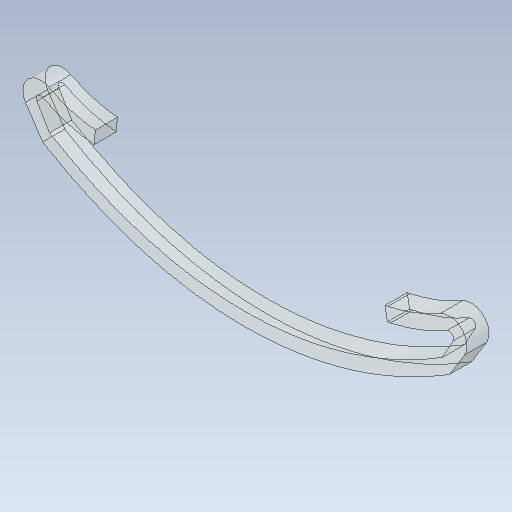
# Autodesk Inventor part: 脚ゴム
Saved by Autodesk Inventor 2020 (Build 240168000, 168)
## iProperties
Created: 2019-11-12
Part Number: 脚ゴム
Material: ゴム、シリコーン
Document SubType Name: Modeling
Designer: tanjihayato
Density: 1.25 g/cm^3
Appearance: クリア
Mass: 2.72773 g
Surface Area: 23.6428 cm^2
Volume: 2.18218 cm^3
Author: tanjihayato
Autodesk Inventor part; units mm, degrees
ref_plane "YZ Plane" through (0, 0, 0) normal (1, 0, 0) x (0, 1, 0)
ref_plane "XZ Plane" through (0, 0, 0) normal (0, 1, 0) x (-1, 0, 0)
ref_plane "XY Plane" through (0, 0, 0) normal (0, 0, 1) x (1, 0, 0)
sketch "スケッチ1" plane through (0, 0, 0) normal (0, 0, 1) x (1, 0, 0)
  arc A0 (47.1325, -53.2266) -> (45.758, -51.8784) centre (46.2557, -52.7457) ccw
  arc A1 (33.009, -56.7784) -> (45.758, -51.8784) centre (23.6069, -13.28) ccw
  arc A2 (11.1932, -28.6204) -> (33.009, -56.7784) centre (28.8377, -37.4801) ccw
  arc A3 (11.1932, -28.6204) -> (-11.1841, -28.6384) centre (0, -23) ccw
  arc A4 (-22.0046, -54.1258) -> (-11.1841, -28.6384) centre (-27.3796, -36.8033) ccw
  arc A5 (-45.6895, -51.9306) -> (-22.0046, -54.1258) centre (-31.2017, -24.4856) ccw
  arc A6 (-45.6895, -51.9306) -> (-47.014, -53.3291) centre (-46.1563, -52.815) ccw
  line L0 (-47.014, -53.3291) -> (-44.145, -58.1151)
  spline S0 degree 4 poles (-44.145, -58.1151) (-43.8381, -58.3003) (-43.4088, -58.5568) (-42.8575, -58.8816) (-42.1841, -59.2711) (-41.6963, -59.5497) (-41.2094, -59.8243) (-40.7232, -60.0949) (-40.2377, -60.3617) (-39.7528, -60.6247) (-39.2684, -60.8839) (-38.7844, -61.1395) (-38.3007, -61.3914) (-37.8172, -61.6398) (-37.334, -61.8846) (-36.8508, -62.1259) (-36.3678, -62.3637) (-35.8847, -62.5981) (-35.4015, -62.8291) (-34.9183, -63.0567) (-34.4349, -63.281) (-33.9513, -63.502) (-33.4675, -63.7196) (-32.9834, -63.934) (-32.499, -64.1451) (-32.0143, -64.3529) (-31.5292, -64.5576) (-31.0437, -64.7589) (-30.5578, -64.9571) (-30.0715, -65.1521) (-29.5847, -65.3439) (-29.0974, -65.5325) (-28.6097, -65.7179) (-28.1214, -65.9001) (-27.6326, -66.0792) (-27.1433, -66.2551) (-26.6534, -66.4278) (-26.163, -66.5974) (-25.6721, -66.7638) (-25.1806, -66.927) (-24.6885, -67.0871) (-24.1958, -67.244) (-23.7026, -67.3978) (-23.2087, -67.5484) (-22.7144, -67.6958) (-22.2194, -67.8401) (-21.7238, -67.9811) (-21.2277, -68.1191) (-20.7311, -68.2538) (-20.2338, -68.3854) (-19.736, -68.5137) (-19.2377, -68.6389) (-18.7388, -68.7609) (-18.2393, -68.8798) (-17.7394, -68.9954) (-17.2389, -69.1078) (-16.7379, -69.217) (-16.2363, -69.323) (-15.7343, -69.4258) (-15.2318, -69.5254) (-14.7289, -69.6218) (-14.2255, -69.7149) (-13.7216, -69.8049) (-13.2173, -69.8915) (-12.7125, -69.975) (-12.2074, -70.0552) (-11.7018, -70.1322) (-11.1959, -70.2059) (-10.6896, -70.2764) (-10.1829, -70.3436) (-9.6759, -70.4075) (-9.1686, -70.4683) (-8.661, -70.5257) (-8.1531, -70.5799) (-7.6449, -70.6308) (-7.1364, -70.6784) (-6.6277, -70.7228) (-6.1188, -70.7639) (-5.6096, -70.8017) (-5.1003, -70.8362) (-4.5907, -70.8674) (-4.0811, -70.8954) (-3.5712, -70.9201) (-3.0613, -70.9415) (-2.5513, -70.9596) (-2.0411, -70.9744) (-1.5309, -70.9859) (-1.0206, -70.9941) (-0.5103, -70.9991) (0, -71.0007) (0.5103, -70.9991) (1.0206, -70.9941) (1.5309, -70.9859) (2.0411, -70.9744) (2.5512, -70.9596) (3.0613, -70.9415) (3.5712, -70.9201) (4.0811, -70.8954) (4.5907, -70.8674) (5.1002, -70.8362) (5.6096, -70.8017) (6.1187, -70.7639) (6.6276, -70.7228) (7.1363, -70.6784) (7.6447, -70.6308) (8.1529, -70.5799) (8.6608, -70.5257) (9.1683, -70.4683) (9.6756, -70.4076) (10.1825, -70.3436) (10.6891, -70.2764) (11.1953, -70.2059) (11.7011, -70.1322) (12.2065, -70.0553) (12.7115, -69.9751) (13.2161, -69.8917) (13.7202, -69.805) (14.2238, -69.7151) (14.727, -69.622) (15.2297, -69.5257) (15.7318, -69.4261) (16.2335, -69.3234) (16.7346, -69.2175) (17.2352, -69.1083) (17.7352, -68.996) (18.2346, -68.8805) (18.7335, -68.7617) (19.2317, -68.6399) (19.7293, -68.5148) (20.2264, -68.3866) (20.7227, -68.2552) (21.2185, -68.1207) (21.7136, -67.983) (22.208, -67.8421) (22.7018, -67.6981) (23.1948, -67.551) (23.6872, -67.4008) (24.1789, -67.2474) (24.6699, -67.0909) (25.1602, -66.9313) (25.6497, -66.7686) (26.1386, -66.6028) (26.6267, -66.4339) (27.1141, -66.2618) (27.6008, -66.0867) (28.0867, -65.9085) (28.5719, -65.7272) (29.0563, -65.5428) (29.54, -65.3554) (30.023, -65.1648) (30.5052, -64.9712) (30.9867, -64.7745) (31.4674, -64.5748) (31.9475, -64.3719) (32.4267, -64.166) (32.9053, -63.9571) (33.3831, -63.745) (33.8603, -63.5299) (34.3367, -63.3117) (34.8124, -63.0904) (35.2875, -62.8661) (35.7619, -62.6386) (36.2356, -62.4081) (36.7086, -62.1745) (37.181, -61.9378) (37.6528, -61.698) (38.124, -61.455) (38.5946, -61.209) (39.0646, -60.9598) (39.5341, -60.7075) (40.003, -60.452) (40.4714, -60.1934) (40.9394, -59.9316) (41.4069, -59.6666) (41.8739, -59.3984) (42.3406, -59.127) (42.8069, -58.8523) (43.4481, -58.4698) (43.9715, -58.1517) (44.3779, -57.9011) (44.6679, -57.7205) knots 0 0 0 0 0 0.014541 0.020333 0.02611 0.031872 0.03762 0.043355 0.049078 0.054789 0.060489 0.066178 0.071857 0.077527 0.083187 0.088839 0.094483 0.10012 0.105749 0.111371 0.116986 0.122595 0.128199 0.133797 0.139389 0.144976 0.150559 0.156136 0.16171 0.167279 0.172845 0.178407 0.183965 0.18952 0.195072 0.20062 0.206166 0.211709 0.21725 0.222788 0.228323 0.233857 0.239388 0.244918 0.250445 0.255971 0.261495 0.267017 0.272538 0.278057 0.283575 0.289092 0.294608 0.300122 0.305635 0.311147 0.316658 0.322169 0.327678 0.333186 0.338694 0.344201 0.349707 0.355213 0.360718 0.366222 0.371726 0.377229 0.382732 0.388235 0.393737 0.399238 0.404739 0.41024 0.415741 0.421241 0.426741 0.432241 0.43774 0.44324 0.448739 0.454238 0.459737 0.465236 0.470734 0.476233 0.481731 0.48723 0.492728 0.498227 0.503725 0.509224 0.514722 0.520221 0.525719 0.531218 0.536717 0.542216 0.547715 0.553214 0.558714 0.564214 0.569713 0.575214 0.580714 0.586215 0.591716 0.597217 0.602718 0.60822 0.613723 0.619225 0.624728 0.630232 0.635736 0.641241 0.646746 0.652251 0.657758 0.663264 0.668772 0.67428 0.679789 0.685299 0.690809 0.69632 0.701832 0.707345 0.712859 0.718374 0.72389 0.729407 0.734925 0.740444 0.745965 0.751487 0.75701 0.762535 0.768061 0.773588 0.779117 0.784648 0.790181 0.795715 0.801252 0.80679 0.812331 0.817873 0.823418 0.828965 0.834515 0.840067 0.845622 0.85118 0.85674 0.862304 0.867871 0.873441 0.879014 0.884591 0.890172 0.895757 0.901345 0.906938 0.912535 0.918137 0.923743 0.929355 0.934971 0.940593 0.946221 0.951854 0.957493 0.963139 0.968791 0.974449 0.980115 0.985788 1 1 1 1 1
  line L1 (44.6679, -57.7205) -> (47.1325, -53.2266)
  arc A7 (4.5969, -37.0887) -> (23.8174, -61.1986) centre (28.8377, -37.4801) ccw
  spline S1 degree 3 poles (23.923, -63.1268) (24.0467, -63.086) (24.1612, -63.0216) (24.3592, -62.8523) (24.4407, -62.7492) (24.5595, -62.5175) (24.5958, -62.3911) (24.6178, -62.1316) (24.6033, -62.0009) (24.5251, -61.7525) (24.4622, -61.6371) (24.3075, -61.4513) (24.2222, -61.3781) (24.0311, -61.2629) (23.9266, -61.2217) (23.8174, -61.1986) knots 0 0 0 0 0.148947 0.148947 0.297893 0.297893 0.44684 0.44684 0.595787 0.595787 0.744733 0.744733 0.872367 0.872367 1 1 1 1
  spline S2 degree 3 poles (23.923, -63.1268) (23.6264, -63.2244) (21.6991, -63.8462) (18.9298, -64.6237) (14.7719, -65.5721) (11.4157, -66.1631) (7.1944, -66.6887) (3.8013, -66.9375) (-0.4475, -67.0324) (-3.8473, -66.9351) (-8.0854, -66.5978) (-11.4616, -66.156) (-15.6527, -65.3916) (-18.978, -64.6118) (-23.0925, -63.431) (-25.7434, -62.5289) (-27.5645, -61.8359) (-27.7718, -61.756) knots -0.770978 -0.770978 -0.770978 -0.770978 -0.760435 -0.70257 -0.673637 -0.615772 -0.58684 -0.528974 -0.500042 -0.442177 -0.413244 -0.355379 -0.326446 -0.268581 -0.239649 -0.181783 -0.174342 -0.174342 -0.174342 -0.174342
  spline S3 degree 3 poles (-27.5161, -59.8282) (-27.6456, -59.8417) (-27.7712, -59.8804) (-28.0006, -60.0037) (-28.1022, -60.0872) (-28.2675, -60.2884) (-28.3298, -60.4042) (-28.4064, -60.6531) (-28.42, -60.7838) (-28.3964, -61.0432) (-28.3594, -61.1693) (-28.2435, -61.3919) (-28.1687, -61.4881) (-27.9885, -61.6491) (-27.8845, -61.7126) (-27.7718, -61.756) knots 0 0 0 0 0.145866 0.145866 0.291731 0.291731 0.437597 0.437597 0.583462 0.583462 0.729328 0.729328 0.864664 0.864664 1 1 1 1
  arc A8 (-27.5161, -59.8282) -> (-20.671, -58.4236) centre (-31.2017, -24.4856) ccw
  arc A9 (-20.671, -58.4236) -> (-4.7434, -37.0245) centre (-27.3796, -36.8033) ccw
  arc A10 (-3.4858, -36.0681) -> (-4.7434, -37.0245) centre (-3.7435, -37.0343) ccw
  arc A11 (-3.4858, -36.0681) -> (3.3494, -36.1037) centre (0, -23) ccw
  arc A12 (4.5969, -37.0887) -> (3.3494, -36.1037) centre (3.597, -37.0726) ccw
  circle A13 centre (0, -23) radius 8.525
  circle A14 centre (0, 0) radius 1.5
  circle A15 centre (-6.3066, -8.8137) radius 1.5
  line L2 (5.2372, 1.6799) -> (11.9265, -19.1744)
  arc A16 (5.2372, 1.6799) -> (-4.7491, 2.7742) centre (0, 0) ccw
  line L3 (-4.7491, 2.7742) -> (-10.1922, -6.5439)
  arc A17 (-10.1922, -6.5439) -> (-10.7715, -8.253) centre (-6.3066, -8.8137) ccw
  line L4 (-10.7715, -8.253) -> (-12.4274, -21.4394)
  arc A18 (11.9265, -19.1744) -> (-12.4274, -21.4394) centre (0, -23) ccw
  arc A19 (-9.0832, -7.6778) -> (-5.0879, -11.555) centre (-6.3066, -8.8137) ccw
  line L5 (-9.0832, -7.6778) -> (-4.9441, 2.4403)
  constraints: 35 point on circle, 20 centre point, 12 end point, 3 tangent, 1 coincident, 1 point on line, 8 other
sketch "スケッチ2" plane through (0, 0, 0) normal (0, 0, 1) x (1, 0, 0)
  spline S0 degree 4 poles (-44.145, -58.1151) (-37.6182, -62.054) (-28.2694, -66.5348) (-15.5407, -70.2705) (0.4425, -71.3509) (16.3869, -70.0942) (29.0453, -66.236) (38.314, -61.6764) (44.6679, -57.7205) knots 0 0 0 0 0 0.314296 0.438586 0.562663 0.686902 1 1 1 1 1
  arc A0 (-45.6895, -51.9306) -> (-47.014, -53.3292) centre (-46.1563, -52.815) ccw
  arc A1 (-45.6895, -51.9306) -> (-34.0657, -55.3875) centre (-31.2017, -24.4856) ccw
  arc A2 (-22.0045, -54.1258) -> (-11.1841, -28.6384) centre (-27.3796, -36.8033) ccw
  arc A3 (32.2678, -56.9238) -> (33.009, -56.7784) centre (28.8377, -37.4801) ccw
  arc A4 (33.009, -56.7784) -> (45.758, -51.8784) centre (23.6069, -13.28) ccw
  arc A5 (47.1325, -53.2266) -> (45.758, -51.8784) centre (46.2557, -52.7457) ccw
  arc A6 (-22.8936, -51.2605) -> (-13.8629, -29.9889) centre (-27.3796, -36.8033) ccw
  arc A7 (-44.289, -49.2776) -> (-33.7888, -52.4003) centre (-31.2017, -24.4856) ccw
  arc A8 (-44.289, -49.2776) -> (-49.5871, -54.8716) centre (-46.1563, -52.815) ccw
  arc A9 (31.7303, -53.9723) -> (32.3752, -53.8461) centre (28.8377, -37.4801) ccw
  arc A10 (32.3752, -53.8461) -> (44.2648, -49.2764) centre (23.6069, -13.28) ccw
  arc A11 (49.7629, -54.6691) -> (44.2648, -49.2764) centre (46.2557, -52.7457) ccw
  line L0 (-49.5871, -54.8716) -> (-45.6951, -60.6836)
  line L1 (46.2535, -60.2673) -> (49.7629, -54.6691)
  line L2 (-33.7888, -52.4003) -> (-34.0657, -55.3875)
  line L3 (-47.014, -53.3292) -> (-44.145, -58.1151)
  line L4 (44.6679, -57.7205) -> (47.1325, -53.2266)
  line L5 (31.7303, -53.9723) -> (32.2678, -56.9238)
  spline S1 degree 5 poles (-45.6951, -60.6836) (-37.3741, -65.7056) (-28.5032, -69.8262) (-19.0469, -72.6542) (0.3831, -75.4348) (19.7882, -72.4725) (29.1916, -69.5658) (38.0209, -65.3927) (46.2535, -60.2673) knots 0 0 0 0 0 0 0.500557 0.500557 0.500557 1 1 1 1 1 1
  point P0 (0, 0)
  point P1 (11.1932, -28.6204)
  point P2 (-33.3656, -63.7642)
  point P3 (-22.3576, -67.7993)
  point P4 (-11.0481, -70.226)
  point P5 (0.4419, -70.9986)
  point P6 (11.9239, -70.0979)
  point P7 (23.204, -67.5475)
  point P8 (34.1337, -63.4043)
  dimension "d0" = 3
  dimension "d1" = 3
  dimension "d2" = 3
  constraints: 24 point on circle, 12 centre point, 12 end point, 13 other
  measures "d1" radial gap between concentric circles of A1 A7
  measures "d2" radial gap between concentric circles of A3 A9
extrude "押し出し1" add sketch "スケッチ2" along normal blind 5
